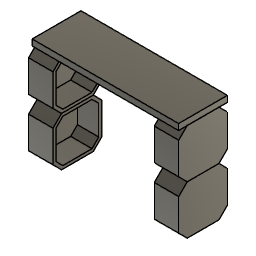
Escritorio v1 (Autodesk Fusion 360 design; units mm, degrees)
Autodesk Fusion 360 part; units mm, degrees
sketch "Boceto1" plane through (0, 0, 0) normal (0, 1, 0) x (1, 0, 0)
  line L0 (1, -2) -> (401, -2)
  line L1 (401, -2) -> (401, -402)
  line L2 (401, -402) -> (1, -402)
  line L3 (1, -402) -> (1, -2)
  dimension "d1" = 400
  dimension "d2" = 400
  constraint horizontal L0
  constraint vertical L1
  constraint horizontal L2
  constraint vertical L3
  measures "d1" distance of L0.start L0.end
  measures "d2" distance of L0.start L2.end
extrude "Extruir1" add sketch "Boceto1" along normal blind 200 makes body 1
chamfer "Chaflán1" distance 70 angle 45 4 edges at (401, 100, 402) (401, 100, 2) (1, 100, 402) (1, 100, 2) on bodies 1
shell "Vaciado1" thickness 25 removed faces 1 at (181, 0, 158.6667) on bodies 1
move_body "Desplazar1" bodies 1 to x (0, -1, 0) y (1, 0, 0) z (0, 0, 1) at (601, 301, 0)
copy_body "CopiarPegarCuerpos1" bodies 1 makes body 2
copy_body "CopiarPegarCuerpos2" bodies 2 1 makes body 3 makes body 4
move_body "Desplazar2" bodies 3 4 to x (1, 0, 0) y (0, 1, 0) z (0, 0, 1) at (0, 0, 400)
copy_body "CopiarPegarCuerpos3" bodies 2 1 makes body 5 makes body 6
move_body "Desplazar3" bodies 5 6 to x (1, 0, 0) y (0, 1, 0) z (0, 0, 1) at (-1000, 0, 0)
copy_body "CopiarPegarCuerpos4" bodies 2 1 makes body 7 makes body 8
move_body "Desplazar4" bodies 7 8 to x (1, 0, 0) y (0, 1, 0) z (0, 0, 1) at (-1000, 0, 400)
sketch "Boceto2" plane through (0, 0, 0) normal (0, 0, 1) x (1, 0, 0)
  line L0 (-400, 300) -> (800, 300)
  line L1 (800, 300) -> (800, -100)
  line L2 (800, -100) -> (-400, -100)
  line L3 (-400, -100) -> (-400, 300)
  constraint horizontal L0
  constraint vertical L1
  constraint horizontal L2
  constraint vertical L3
extrude "Extruir2" add sketch "Boceto2" against normal blind 50 separate body makes body 9
move_body "Desplazar5" bodies 9 to x (1, 0, 0) y (0, 1, 0) z (0, 0, 1) at (0, 0, 850)
move_body "Desplazar6" bodies 7 5 6 8 to x (-1, 0, 0) y (0, -1, 0) z (0, 0, 1) at (-598, -130, 0)
move_body "Desplazar7" bodies 6 8 5 7 to x (1, 0, 0) y (0, 1, 0) z (0, 0, 1) at (0, 300, 0)
